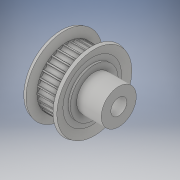
# Autodesk Inventor part: GPA30GT2060-B-H5_b
Saved by Autodesk Inventor 2019 (Build 230136000, 136)
## iProperties
Created: 2023-11-19
Part Number: GPA30GT2060-B-H5_b
Material: Generic
Catalog Web Link: www.cadenas.de
Description: GPA_GT2040, GPA_GT2060, GPA_GT2090, KGPA_GT2040, KGPA_GT2060, KGPA_GT2090, KGPK_GT2040, KGPK_GT2060, KGPK_GT2090_body-High Torque Timing Pulleys 2GT Type
Vendor: MISUMI
Document SubType Name: Modeling
Designer: psAdmin
Manufacturer: MISUMI
Mass: 3.23564 g
Surface Area: 25.902 cm^2
Volume: 3.23564 cm^3
Density: 1 g/cm^3
Appearance: PSOLRGB-175-175-175
Category: PARTsolutions
Company: MISUMI
Title: GPA30GT2060-B-H5
Author: Cadenas PARTsolutions
Comments: High Torque Timing Pulleys 2GT Type
PSOL_IDENT_0: {$CADENAS_DATA/23d-libs/misumi/metric/51_timing_pulleys/gpa__gt2/gpa_gt2.prj},477 {VTYP=3D},{NB=GPA3
PSOL_IDENT_1: 0GT2060-B-H5_b},{LINA=GPA30GT2060-B-H5},{NN=GPA_GT2040, GPA_GT2060, GPA_GT2090, KGPA_GT2040, KGPA_GT
PSOL_IDENT_2: 2060, KGPA_GT2090, KGPK_GT2040, KGPK_GT2060, KGPK_GT2090_body},{DATE=25.04.2022 01:22:58},{GEOMDATE=
PSOL_IDENT_3: 22.12.2021 00:45:33},{VERSION=},{LINEID=110},{WBVAR=MAT,ST,TNW,PS,SBS,DD,Z,J,Q,R,S,T,ALT1,ALT2,M,QSC
PSOL_IDENT_4: ,QFC,QTC,ALT3,K,KSC,KFC,KTC,ALT4,ZM,ZSC,ZFC,ZTC,ALT5,BC,ALT6,ALT7,ALT8,FC,ALT13,BN},{WBNUMERIC=DD,Z,
PSOL_IDENT_5: J,Q,R,S,T,QSC,QFC,QTC,K,KSC,KFC,KTC,ZSC,ZFC,ZTC,BC,FC,BN}  {NB=GPA30GT2060-B-H5_b},{LINA=GPA30GT2060
PSOL_IDENT_6: -B-H5},{KT=DUMMY},{PN=GPA30GT2060-B-H5},{TYPE=GPA},{MAT=AA},{ST=CA},{NT=30},{TNW=GT2060},{BW=6},{A=7
PSOL_IDENT_7: .0},{W=10.3},{L=18.0},{PS=B},{PSA= 'A','B' },{SBS=H},{SBSALG= 'H','Round Hole','V','Stepped Hole','F'
PSOL_IDENT_8: ,'Stepped Hole (Counterbore holes on the boss side)' },{DD=5.00},{DDALG=[5:6/1],[6.35],[7:8/1]},{DDH
PSOL_IDENT_9: A=[5:6/1],[6.35],[7:11/1]},{DDHB=[5:6/1],[6.35],[7:8/1]},{DDPA=},{DDPB=},{DDNA=},{DDNB=},{DDNKA=0},{
PSOL_IDENT_10: DDNKB=0},{DDVA=[5:6/1],[6.35],[7:9/1]},{DDVFB=[5:5/1]},{DDYA=[5:9/1]},{Z=0},{ZALG=0},{ZMIN=7},{ZAMAX=
PSOL_IDENT_11: 11},{ZBMAX=7},{J=0.0},{JALG=0},{JMAX=16},{Q=0},{R=0},{QRALG=0},{QRMIN=7},{QRMAX=11},{S=0.0},{SALG=0}
PSOL_IDENT_12: ,{SMAX=4.300},{T=0.0},{TALG=0},{TMAX=5.000},{PD=19.10},{OD=18.59},{D=11},{DE=11},{DDZ=5},{F=24},{E=1
PSOL_IDENT_13: 5},{BB=0},{TT=0},{M1=3},{AC=-},{ALT1=},{ALT1A= '','Not applicable' },{ANG=120},{ALT2=},{ALT2A= '','N
PSOL_IDENT_14: ot applicable' },{M=N/A},{MALG= 'N/A' },{MM=0.000},{MPHD=0.000},{MA= 'N/A' },{MSA= 'N/A' },{QSC=0.0}
PSOL_IDENT_15: ,{QSCA=0},{QFC=0.0},{QFCA=0},{QTC=0.0},{QTCA=0},{QPCDMIN=9},{QPCDMINALG=9},{QPCDMAX=7},{ALT2PN=},{AL
PSOL_IDENT_16: T3=},{ALT3A= '','Not applicable' },{K=0.0},{KA=0},{KAMIN=4},{KAMAX=0},{KSMAX=0},{KSC=0.0},{KSCA=0},{
PSOL_IDENT_17: KFC=0.0},{KFCA=0},{KTC=0.0},{KTCA=0},{KSCMIN=9.000},{KPCDMIN=9.000},{KPCDMINALG=13.000},{KPCDMAX=7.0
PSOL_IDENT_18: 00},{ALT3PN=},{ALT4=},{ALT4ALG= '','Not applicable' },{ALT4MIN=15.500},{ALT4MAX=3.500},{ZM=N/A},{ZMA
PSOL_IDENT_19: LG= 'N/A' },{ZMFTALG= 'N/A' },{ZMSALG= 'N/A' },{ZMDD1=0.0},{ZMDD2=0.0},{ZMHH=0.0},{ZSC=0.0},{ZSCALG=
PSOL_IDENT_20: [0]},{ZFC=0.0},{ZFCALG=[0]},{ZTC=0.0},{ZTCALG=[0]},{ZPCDMIN=0.000},{ZPCDMINALG=0.000},{ZPCDMAX=7.000
PSOL_IDENT_21: },{ALT4PN=},{ALT5=},{ALT5ALG= '','w/o BC (Boss Cut)','-BC','with BC (Boss Cut)' },{ALT5PN=},{BC=0.0}
PSOL_IDENT_22: ,{BCALG=0},{BCMIN=3.000},{BCMAX=7.700},{ALT6=},{ALT7=},{ALT7ALG= '','w/o Flange Attached on One Side
PSOL_IDENT_23: Only','-RFC','with RFC (Flange Attached on The Boss Side Only)','-LFC','with LFC (Flange Attached o
PSOL_IDENT_24: n The Opposite Side Only)' },{ALT8=},{ALT8ALG='','w/o FC (Flange Cut)','-FC','with FC (Flange Cut)'}
PSOL_IDENT_25: ,{ALT8PN=},{FC=0.0},{FCA=0},{ODAINT=22.000},{FCMIN=20},{FCMAX=22},{WLBC=18},{SL=2.5},{SL2=2.5},{KTT=
PSOL_IDENT_26: 2.5},{KYY=3},{TAP=0},{MATALG= 'AA','Aluminum Alloy 2000 series' , '6000','6000 Series Aluminum Alloy'
PSOL_IDENT_27: },{STALG= 'CA','Clear Anodize' },{ALT13=},{BN=0.000},{BNMIN=8.200},{BNMAX=17.700},{ALT13ALG= '','w/
PSOL_IDENT_28: o BN (Hub Lengthening)','BN','with BN (Hub Lengthening)' },{BNALG=0},{BNPN=}
NB: GPA30GT2060-B-H5_b
NN: GPA_GT2040, GPA_GT2060, GPA_GT2090, KGPA_GT2040, KGPA_GT2060, KGPA_GT2090, KGPK_GT2040, KGPK_GT2060, KGPK_GT2090_body
NT: 30
NBSYN: $PN._b
LINA: GPA30GT2060-B-H5
CATALOG: Misumi
PN: GPA30GT2060-B-H5
MAT: Aluminum Alloy 2000 series
ST: Clear Anodize
TNW: GT2060
A: 7
W: 10.3
L: 18
PS: B
SBS: Round Hole
DD: 5
Z: 0
J: 0
Q: 0
R: 0
S: 0
T: 0
PD: 19.1
OD: 18.59
D: 11
F: 24
E: 15
AC: -
ALT1: Not applicable
ALT2: Not applicable
M: N/A
QSC: 0
QFC: 0
QTC: 0
ALT3: Not applicable
K: 0
KSC: 0
KFC: 0
KTC: 0
ALT4: Not applicable
ZM: N/A
ZMDD1: 0
ZMDD2: 0
ZMHH: 0
ZSC: 0
ZFC: 0
ZTC: 0
ALT5: w/o BC (Boss Cut)
BC: 0
ALT6: w/o Flange not Attached
ALT7: w/o Flange Attached on One Side Only
ALT8: w/o FC (Flange Cut)
FC: 0
ALT13: w/o BN (Hub Lengthening)
BN: 0
SUPPLIER: MISUMI
ARTICLENO: GPA30GT2060-B-H5_b
BOMINFO: GPA30GT2060-B-H5
CREATOR: CADENAS GmbH
Autodesk Inventor part; units mm, degrees
ref_plane "YZ Plane" through (0, 0, 0) normal (1, 0, 0) x (0, 1, 0)
ref_plane "XZ Plane" through (0, 0, 0) normal (0, 1, 0) x (-1, 0, 0)
ref_plane "XY Plane" through (0, 0, 0) normal (0, 0, 1) x (1, 0, 0)
sketch "Sketch_17" plane through (0, 0, 0) normal (0, 0, 1) x (1, 0, 0)
  line L0 (12.85, 0) -> (-5.15, 0)
  line L1 (-5.15, 0) -> (-5.15, 7.5)
  line L2 (-5.15, 7.5) -> (-3.5, 7.5)
  line L3 (-3.5, 7.5) -> (-3.5, 9.295)
  line L4 (-3.5, 9.295) -> (3.5, 9.295)
  line L5 (3.5, 9.295) -> (3.5, 7.5)
  line L6 (3.5, 7.5) -> (5.15, 7.5)
  line L7 (5.15, 7.5) -> (5.15, 5.5)
  line L8 (5.15, 5.5) -> (12.85, 5.5)
  line L9 (12.85, 5.5) -> (12.85, 0)
  line L10 (12.85, 0) -> (-5.15, 0)
  constraints: 22 end point
revolve "Revolution1" add sketch "Sketch_17" angle 360 about axis through (12.85, 0, 0) along (1, 0, 0)
sketch "Sketch_18" plane through (0, 0, 0) normal (1, 0, 0) x (0, 1, 0)
  line L0 (9.5025, 0.9509) -> (9.2507, 0.9257)
  line L1 (9.2507, 0.9257) -> (9.2621, 0.7934)
  arc A0 (9.1605, 0.6723) -> (9.2621, 0.7934) centre (9.1505, 0.7838) ccw
  arc A1 (9.1605, 0.6723) -> (9.1605, -0.6723) centre (9.221, 0) ccw
  arc A2 (9.2621, -0.7934) -> (9.1605, -0.6723) centre (9.1505, -0.7838) ccw
  line L2 (9.2621, -0.7934) -> (9.2507, -0.9257)
  line L3 (9.2507, -0.9257) -> (9.5025, -0.9509)
  arc A3 (9.5025, -0.9509) -> (9.5025, 0.9509) centre (0, 0) ccw
  constraints: 8 end point, 8 point on circle, 4 centre point
extrude "Extrusion1" cut sketch "Sketch_18" along normal mid plane 7
pattern_circular "Circular Pattern1" count 30 over 360 about axis through (0, 0, 0) along (1, 0, 0) of "Extrusion1"
sketch "Sketch_20" plane through (0, 0, 0) normal (0, 0, 1) x (1, 0, 0)
  line L0 (50, 0) -> (-50, 0)
  line L1 (3.5, 9.295) -> (3.5, 7.5)
  line L2 (3.5, 7.5) -> (4.5, 7.5)
  line L3 (4.5, 7.5) -> (4.5, 9.1633)
  line L4 (4.5, 9.1633) -> (5.1907, 11.7412)
  line L5 (5.1907, 11.7412) -> (4.2248, 12)
  line L6 (4.2248, 12) -> (3.5, 9.295)
  constraints: 14 end point
revolve "Revolution2" add sketch "Sketch_20" angle 360 about axis through (50, 0, 0) along (1, 0, 0)
sketch "Sketch_21" plane through (0, 0, 0) normal (0, 0, 1) x (1, 0, 0)
  line L0 (50, 0) -> (-50, 0)
  line L1 (-5.1907, 11.7412) -> (-4.5, 9.1633)
  line L2 (-4.5, 9.1633) -> (-4.5, 7.5)
  line L3 (-4.5, 7.5) -> (-3.5, 7.5)
  line L4 (-3.5, 7.5) -> (-3.5, 9.295)
  line L5 (-3.5, 9.295) -> (-4.2248, 12)
  line L6 (-4.2248, 12) -> (-5.1907, 11.7412)
  constraints: 14 end point
revolve "Revolution3" add sketch "Sketch_21" angle 360 about axis through (50, 0, 0) along (1, 0, 0)
sketch "Sketch5" plane through (12.85, 0, 0) normal (1, 0, 0) x (0, 0, -1)
  point P0 (0, 0)
hole "Hole1" at (12.85, 0, 0) direction (-1, 0, 0) diameter 5 depth 18
body "Solid1"
